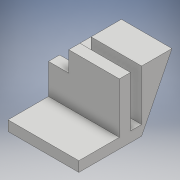
# Autodesk Inventor part: Ooze_Ramp_Top
Saved by Autodesk Inventor 2017 (Build 210142000, 142)
## iProperties
Created: 2017-01-16
Part Number: Ooze_Ramp_Top
Material: Generic
Document SubType Name: Modeling
Designer: willt
Density: 1 g/cm^3
Appearance: Default
Author: willt
Autodesk Inventor part; units mm, degrees
ref_plane "YZ Plane" through (0, 0, 0) normal (1, 0, 0) x (0, 1, 0)
ref_plane "XZ Plane" through (0, 0, 0) normal (0, 1, 0) x (-1, 0, 0)
ref_plane "XY Plane" through (0, 0, 0) normal (0, 0, 1) x (1, 0, 0)
sketch "Sketch1" plane through (0, 0, 0) normal (1, 0, 0) x (0, 1, 0)
  line L0 (0, 0) -> (10, 0)
  line L1 (10, 0) -> (0, -20)
  line L2 (0, -20) -> (0, 0)
  dimension "d0" = 20
  dimension "d1" = 10
  constraints: 6 end point, 1 horizontal, 1 perpendicular
  measures "d0" distance of L1.end L0.start
  measures "d1" distance of L0.start L0.end
extrude "Extrusion1" add sketch "Sketch1" along normal blind 35
sketch "Sketch7" plane through (0, 0, -20) normal (0, -1, 0) x (1, 0, 0)
  line L0 (35, 20) -> (35, 0) projected
  line L1 (0, 0) -> (0, 20) projected
  line L2 (35, 0) -> (0, 0)
  line L3 (0, 0) -> (0, 5)
  line L4 (0, 5) -> (35, 5)
  line L5 (35, 5) -> (35, 0)
  dimension "d17" = 5
  constraints: 8 end point, 2 parallel, 1 horizontal, 1 perpendicular, 1 point on line
  measures "d17" distance of L2.end L3.end
extrude "Extrusion7" add sketch "Sketch7" along normal blind 11
sketch "Sketch8" plane through (0, 0, -15) normal (0, 0, 1) x (1, 0, 0)
  line L0 (35, -11) -> (0, -11)
  line L1 (0, -11) -> (0, -5.5)
  line L2 (0, -5.5) -> (35, -5.5)
  line L3 (35, -5.5) -> (35, -11)
  point P0 (0, 0)
  dimension "d20" = 5.5
  dimension "d26" = 35
  constraints: 8 end point, 2 parallel, 1 horizontal, 1 perpendicular
  measures "d20" distance of L0.end L1.end
  measures "d26" distance of L1.end L2.end
extrude "Extrusion8" add sketch "Sketch8" along normal blind 15
sketch "Sketch9" plane through (0, -11, -20) normal (0, -1, 0) x (1, 0, 0)
  line L0 (0, 5) -> (0, 20) projected
  line L1 (35, 0) -> (0, 0)
  line L2 (0, 0) -> (0, 5)
  line L3 (0, 5) -> (35, 5)
  line L4 (35, 5) -> (35, 0)
  dimension "d23" = 5
  constraints: 8 end point, 2 parallel, 1 horizontal, 1 perpendicular
  measures "d23" distance of L1.end L0.start
extrude "Extrusion9" add sketch "Sketch9" along normal blind 20
sketch "Sketch10" plane through (35, 0, 0) normal (1, 0, 0) x (0, 0, -1)
  line L0 (15, 0) -> (0, 0) projected
  line L1 (0, 0) -> (-10, 0)
  line L2 (0, -11) -> (-10, -11)
  line L3 (-10, -11) -> (-10, -5.5)
  line L4 (-10, -5.5) -> (0, -5.5)
  line L5 (0, -5.5) -> (0, -11)
  line L6 (0, 10) -> (20, 0) projected
  line L7 (0, 10) -> (-10, 15)
  line L8 (20, 0) -> (0, 10) projected
  line L9 (-10, 0) -> (-10, 15)
  line L10 (0, 0) -> (0, 10) projected
  line L11 (0, 0) -> (0, 10)
  dimension "d27" = 10
  dimension "d30" = 10
  constraints: 16 end point, 2 collinear, 2 horizontal, 2 parallel, 1 perpendicular, 1 vertical
  measures "d27" distance of L0.end L1.end
  measures "d30" distance of L3.end L4.end
extrude "Extrusion10" add sketch "Sketch10" against normal blind 25
body "Solid1"
